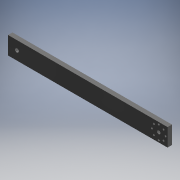
# Autodesk Inventor part: bar arms
Saved by Autodesk Inventor 2019 (Build 230136000, 136)
## iProperties
Part Number: bar arms
Material: Generic
Document SubType Name: Modeling
Designer: Delta
Appearance: Default
Author: Delta
Autodesk Inventor part; units mm, degrees
ref_plane "YZ Plane" through (0, 0, 0) normal (1, 0, 0) x (0, 1, 0)
ref_plane "XZ Plane" through (0, 0, 0) normal (0, 1, 0) x (-1, 0, 0)
ref_plane "XY Plane" through (0, 0, 0) normal (0, 0, 1) x (1, 0, 0)
sketch "Sketch1" plane through (0, 0, 0) normal (0, 0, 1) x (1, 0, 0)
  line L0 (0, 0) -> (228.6, 0)
  line L1 (228.6, 0) -> (228.6, 25.4)
  line L2 (228.6, 25.4) -> (0, 25.4)
  line L3 (0, 25.4) -> (0, 0)
  dimension "d0" = 228.6
  dimension "d1" = 25.4
  constraints: 8 end point, 2 parallel, 1 horizontal, 1 perpendicular
  measures "d0" distance of L2.end L1.end
  measures "d1" distance of L1.end L0.end
extrude "Extrusion1" add sketch "Sketch1" along normal blind 6.35
sketch "Sketch2" plane through (0, 0, 6.35) normal (0, 0, 1) x (1, 0, 0)
  line L0 (0, 25.4) -> (0, 0) projected
  line L1 (0, 0) -> (228.6, 0) projected
  line L2 (228.6, 25.4) -> (0, 25.4) projected
  circle A0 centre (12.7, 12.7) radius 2.8829
  dimension "d4" = 12.7
  dimension "d5" = 25.4
  dimension "d6" = 5.7658
  dimension "d15" = 12.7
  constraints: 1 centre point, 1 coincident
  measures "d4" distance from line of L0 point (12.7, 12.7)
  measures "d5" distance between parallel lines of L1 L2
  measures "d6" diameter of A0
  measures "d15" distance from line of L2 A0.centre
extrude "Extrusion2" cut sketch "Sketch2" against normal through all
sketch "Sketch3" plane through (0, 0, 6.35) normal (0, 0, 1) x (1, 0, 0)
  line L0 (0, 0) -> (228.6, 0) projected
  line L1 (228.6, 25.4) -> (0, 25.4) projected
  line L2 (228.6, 0) -> (228.6, 25.4) projected
  circle A0 centre (215.9, 12.7) radius 2.54
  dimension "d9" = 25.4
  dimension "d10" = 12.7
  dimension "d11" = 12.7
  dimension "d12" = 5.08
  constraints: 1 centre point, 1 coincident
  measures "d9" distance between parallel lines of L0 L1
  measures "d10" distance from line of L2 point (215.9, 12.7)
  measures "d11" distance from line of L1 point (215.9, 12.7)
  measures "d12" diameter of A0
extrude "Extrusion3" cut sketch "Sketch3" against normal through all
sketch "Sketch4" plane through (0, 0, 6.35) normal (0, 0, 1) x (1, 0, 0)
  circle A0 centre (215.9, 12.7) radius 2.54 projected
  circle A1 centre (215.9, 12.7) radius 9.779
  line L0 (215.9, 22.479) -> (208.9787, 19.6083)
  line L1 (208.9787, 19.6083) -> (206.121, 12.7)
  line L2 (206.121, 12.7) -> (208.9917, 5.7787)
  line L3 (208.9917, 5.7787) -> (215.9, 2.921)
  line L4 (215.9, 2.921) -> (222.8213, 5.7917)
  line L5 (222.8213, 5.7917) -> (225.679, 12.7)
  line L6 (225.679, 12.7) -> (222.8083, 19.6213)
  line L7 (222.8083, 19.6213) -> (215.9, 22.479)
  circle A2 centre (215.9, 22.479) radius 1.3589
  circle A3 centre (222.8083, 19.6213) radius 1.3589
  circle A4 centre (225.679, 12.7) radius 1.3589
  circle A5 centre (222.8213, 5.7917) radius 1.3589
  circle A6 centre (215.9, 2.921) radius 1.3589
  circle A7 centre (208.9917, 5.7787) radius 1.3589
  circle A8 centre (206.121, 12.7) radius 1.3589
  circle A9 centre (208.9787, 19.6083) radius 1.3589
  point P0 (0, 0)
  dimension "d16" = 19.558
  dimension "d17" = 7.493
  dimension "d18" = 2.7178
  dimension "d19" = 2.7178
  dimension "d20" = 2.7178
  dimension "d21" = 2.7178
  dimension "d22" = 2.7178
  dimension "d23" = 2.7178
  dimension "d24" = 2.7178
  dimension "d25" = 2.7178
  constraints: 16 end point, 9 coincident, 8 centre point, 6 perpendicular, 10 other
  measures "d17" distance of L0.start L0.end
  measures "d18" diameter of A2
  measures "d19" diameter of A8
  measures "d20" diameter of A7
  measures "d21" diameter of A6
  measures "d22" diameter of A5
  measures "d23" diameter of A4
  measures "d24" diameter of A3
  measures "d25" diameter of A9
extrude "Extrusion4" cut sketch "Sketch4" against normal through all contours L6 A4 A1 | A1 A4 | A1 A4 L5 | L5 A4 L6 | A3 L6 A1 | A1 A3 | A5 A1 | A1 L5 A5 | L5 L4 A5 | A3 L7 L6 | L7 A3 A1 | A1 A5 L4 | A6 A1 L4 | L4 L3 A6 | A2 L0 L7 | L7 A1 A2 | A1 A2 | A6 A1 | A1 A6 L3 | L0 A2 A1 | A7 A1 L3 | L3 L2 A7 | A9 L1 L0 | L0 A1 A9 | A7 A1 | A1 A7 L2 | A1 A9 | L1 A9 A1 | A8 A1 | A1 L2 A8 | L2 L1 A8 | A8 L1 A1
equation "\"d4\" = 0.5 * d5"
equation "\"d15\" = 0.5 * d5"
equation "\"d10\" = 0.5 * d9"
equation "\"d11\" = 0.5 * d9"
equation "\"d19\" = d18"
equation "\"d20\" = d18"
equation "\"d21\" = d18"
equation "\"d22\" = d18"
equation "\"d23\" = d18"
equation "\"d24\" = d18"
equation "\"d25\" = d18"
body "Solid1"
